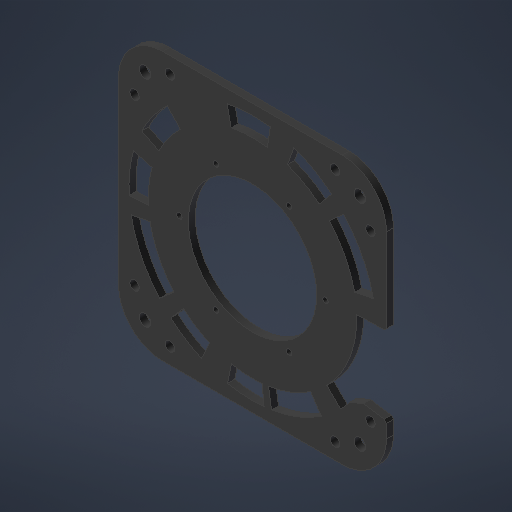
# Autodesk Inventor part: stator_mount_01_alu
Saved by Autodesk Inventor 2026.1 (Build 301233000, 233)
## iProperties
Created: 2026-04-12
Part Number: stator_mount_01_alu
Material: Generic
Document SubType Name: Modeling
Designer: aaron
Density: 1 g/cm^3
Appearance: Default
Author: aaron
Autodesk Inventor part; units mm, degrees
ref_plane "YZ Plane" through (0, 0, 0) normal (1, 0, 0) x (0, 1, 0)
ref_plane "XZ Plane" through (0, 0, 0) normal (0, 1, 0) x (-1, 0, 0)
ref_plane "XY Plane" through (0, 0, 0) normal (0, 0, 1) x (1, 0, 0)
sketch "Sketch1" plane through (0, 0, 0) normal (0, 0, 1) x (1, 0, 0)
  circle A0 centre (0, 0) radius 29
  circle A1 centre (0, 0) radius 60.5
  line L0 (-40.5, 60.5) -> (40.5, 60.5)
  line L1 (60.5, 40.5) -> (60.5, -40.5)
  line L2 (40.5, -60.5) -> (-40.5, -60.5)
  line L3 (-60.5, -40.5) -> (-60.5, 40.5)
  arc A2 (-40.5, 60.5) -> (-60.5, 40.5) centre (-40.5, 40.5) ccw
  arc A3 (60.5, 40.5) -> (40.5, 60.5) centre (40.5, 40.5) ccw
  arc A4 (40.5, -60.5) -> (60.5, -40.5) centre (40.5, -40.5) ccw
  arc A5 (-60.5, -40.5) -> (-40.5, -60.5) centre (-40.5, -40.5) ccw
  dimension "d0" = 58
  dimension "d1" = 121
  dimension "d2" = 20
  constraints: 12 tangent, 8 end point, 8 point on circle, 6 centre point, 3 equal radius, 2 coincident, 2 parallel, 1 horizontal, 1 perpendicular
  measures "d0" diameter of A0
  measures "d1" diameter of A1
  measures "d2" radius of A2
extrude "Extrusion1" add sketch "Sketch1" along normal blind 3.18
sketch "Sketch4" plane through (0, 0, 3.18) normal (0, 0, 1) x (1, 0, 0)
  circle A0 centre (0, 0) radius 51.5771
  circle A1 centre (0, 0) radius 43.9861
  circle A2 centre (0, 0) radius 55.7776
  circle A3 centre (0, 0) radius 47.0962
  circle A4 centre (0, 0) radius 42.5777
  circle A5 centre (0, 0) radius 45.3862
  line L0 (0, 0) -> (8.4363, 58.2297)
  line L1 (0, 0) -> (-12.4381, 59.4602)
  line L2 (0, 0) -> (20.1214, 56.5368)
  line L3 (0, 0) -> (38.2622, 45.8865)
  line L4 (0, 0) -> (43.6183, 40.0538)
  line L5 (0, 0) -> (57.1725, 11.9596)
  line L6 (0, 0) -> (57.4745, 1.6902)
  line L7 (0, 0) -> (41.5878, -40.9399)
  line L8 (0, 0) -> (-40.6993, 42.5777)
  line L9 (0, 0) -> (-51.5874, 25.3844)
  line L10 (0, 0) -> (-57.9992, 16.3021)
  line L11 (0, 0) -> (-60.0133, -3.6073)
  line L12 (0, 0) -> (-59.5436, -11.4224)
  line L13 (0, 0) -> (-44.1098, -38.6301)
  line L14 (0, 0) -> (-38.6281, -43.7925)
  line L15 (0, 0) -> (-24.369, -53.7638)
  line L16 (0, 0) -> (-11.9508, -58.1405)
  line L17 (0, 0) -> (5.5489, -59.3314)
  line L18 (0, 0) -> (37.2684, -55.5197)
  line L19 (0, 0) -> (10.7128, -68.7832)
  point P0 (-50.0468, 24.6263)
  point P1 (-42.2573, 20.7934)
  point P2 (-32.5426, 34.0445)
  point P3 (-38.5413, 40.3201)
  point P4 (-55.6771, -3.3466)
  point P5 (-47.0113, -2.8257)
  point P6 (-45.3392, 12.7437)
  point P7 (-53.6968, 15.0928)
  point P8 (-41.9609, -36.7481)
  point P9 (-35.4299, -31.0285)
  point P10 (-46.2528, -8.8728)
  point P11 (-54.7788, -10.5083)
  point P12 (-23.0268, -50.8026)
  point P13 (-19.4428, -42.8955)
  point P14 (-31.1542, -35.3194)
  point P15 (-36.897, -41.83)
  point P16 (5.1939, -55.5352)
  point P17 (4.3855, -46.8915)
  point P18 (-9.4824, -46.1317)
  point P19 (-11.2303, -54.6353)
  point P20 (8.5837, -55.1131)
  point P21 (31.0871, -46.3113)
  point P22 (26.2486, -39.1032)
  point P23 (7.2477, -46.5351)
  point P24 (33.5624, -33.0395)
  point P25 (39.7491, -39.1298)
  point P26 (55.7535, 1.6396)
  point P27 (47.0758, 1.3844)
  point P28 (46.0984, 9.6431)
  point P29 (54.5959, 11.4206)
  point P30 (41.0837, 37.7263)
  point P31 (34.6892, 31.8544)
  point P32 (30.1611, 36.1712)
  point P33 (35.7209, 42.8387)
  point P34 (18.702, 52.5488)
  point P35 (15.7912, 44.3699)
  point P36 (7.9975, 55.2013)
  point P37 (-11.4206, 54.5959)
  point P38 (-9.6431, 46.0984)
  point P39 (6.7528, 46.6095)
  dimension "d76" = 103.1542
  dimension "d78" = 94.1923
  constraints: 40 end point, 6 centre point, 6 coincident
  measures "d76" diameter of A0
  measures "d78" diameter of A3
extrude "Extrusion4" cut sketch "Sketch4" against normal through all contours A0 L7 A3 L6 | A0 L6 A2 L7 | L5 A3 L4 A0 | A0 L4 A2 L5 | L18 A2 L19 A0 | A0 L19 A3 L18 | L3 A3 L2 A0 | A0 L2 A2 L3 | L17 A2 L16 A0 | A0 L16 A3 L17 | L0 A3 L1 A0 | A0 L1 A2 L0 | L15 A2 L14 A0 | A0 L14 A3 L15 | L8 A3 L9 A0 | A0 L9 A2 L8 | L13 A2 L12 A0 | A0 L12 A3 L13 | L10 A3 L11 A0 | A0 L11 A2 L10
sketch "Sketch5" plane through (0, 0, 3.18) normal (0, 0, 1) x (1, 0, 0)
  circle A0 centre (-48.5, -48.5) radius 2.65
  circle A1 centre (-48.5, 48.5) radius 2.65
  circle A2 centre (48.5, -48.5) radius 2.65
  circle A3 centre (48.5, 48.5) radius 2.65
  circle A4 centre (0, 0) radius 29 projected
  circle A5 centre (0, 0) radius 33
  circle A6 centre (-33, 0) radius 1.25
  circle A7 centre (-16.5, -28.5788) radius 1.25
  circle A8 centre (16.5, -28.5788) radius 1.25
  circle A9 centre (33, 0) radius 1.25
  circle A10 centre (0, 0) radius 65
  line L0 (0, 0) -> (-48.5, -48.5)
  line L1 (0, 0) -> (-46.4652, -66.3592)
  line L2 (0, 0) -> (-57.2887, -40.114)
  circle A11 centre (-37.2825, -53.2449) radius 2.15
  circle A12 centre (-53.2449, -37.2825) radius 2.15
  circle A13 centre (53.2449, -37.2825) radius 2.15
  circle A14 centre (37.2825, -53.2449) radius 2.15
  circle A15 centre (37.2825, 53.2449) radius 2.15
  circle A16 centre (53.2449, 37.2825) radius 2.15
  circle A17 centre (-53.2449, 37.2825) radius 2.15
  circle A18 centre (-37.2825, 53.2449) radius 2.15
  circle A19 centre (16.5, 28.5788) radius 1.25
  circle A20 centre (-16.5, 28.5788) radius 1.25
  dimension "d61" = 66
  dimension "d57" = 5.3
  dimension "d58" = 5.3
  dimension "d59" = 5.3
  dimension "d60" = 5.3
  dimension "d62" = 2.5
  dimension "d65" = 360
  dimension "d67" = 130
  dimension "d68" = 10
  dimension "d69" = 10
  dimension "d70" = 4.3
  dimension "d71" = 4.3
  dimension "d74" = 360
  constraints: 19 centre point, 6 end point, 2 coincident, 2 point on circle, 2 point on line, 1 horizontal alignment, 32 other
  measures "d57" diameter of A0
  measures "d58" diameter of A1
  measures "d59" diameter of A3
  measures "d60" diameter of A2
  measures "d62" diameter of A6
  measures "d67" diameter of A10
  measures "d68" angle of L0 L1
  measures "d69" angle of L2 L0
  measures "d70" diameter of A11
  measures "d71" diameter of A12
extrude "Extrusion5" cut sketch "Sketch5" against normal through all contours A0 | A1 | A2 | A3 | A6 A5 | A5 A6 | A12 A10 L2 | L2 A10 A12 | A7 A5 | A5 A7 | A11 A10 L1 | L1 A10 A11 | L2 A12 A10 | A10 A12 L2 | L1 A11 A10 | A10 A11 L1 | A20 A5 | A5 A20 | A17 A10 | A10 A17 | A8 A5 | A5 A8 | A14 A10 | A10 A14 | A19 A5 | A5 A19 | A18 A10 | A10 A18 | A9 A5 | A5 A9 | A13 A10 | A10 A13 | A15 A10 | A10 A15 | A16 A10 | A10 A16
sketch "Sketch6" plane through (0, 0, 3.18) normal (0, 0, 1) x (1, 0, 0)
  arc A0 (39.7491, -39.1298) -> (55.7535, 1.6396) centre (0, 0) ccw projected
  line L0 (64.1152, -33.9991) -> (64.1152, 1.6396)
  line L1 (55.7535, 1.6396) -> (64.1152, 1.6396)
  line L2 (64.1152, -33.9991) -> (46.2085, -31.2396)
  point P0 (47.5954, -29.0829)
  point P1 (55.585, -4.6304)
  constraints: 6 end point, 3 point on circle, 1 horizontal, 1 vertical
extrude "Extrusion6" cut sketch "Sketch6" against normal through all
chamfer "Chamfer2" distance 4 angle 45 1 edges at (46.2085, -31.2396, 1.59)
chamfer "Chamfer3" distance 1 angle 45 2 edges at (60.5, 1.6396, 1.59) (60.5, -33.4419, 1.59)
equation "\"d58\" = d57"
equation "\"d59\" = d57"
equation "\"d60\" = d57"
equation "\"d69\" = d68"
body "Solid1"
